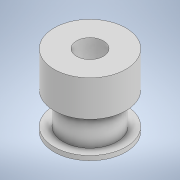
# Autodesk Inventor part: 20T pulley 6 mm bore GT2
Saved by Autodesk Inventor 2022 (Build 260153000, 153)
## iProperties
Created: 2022-08-12
Part Number: 20T pulley 6 mm bore GT2
Material: Genérico
Document SubType Name: Modeling
Designer: JK
Density: 1 g/cm^3
Appearance: Valor por defecto
Author: JK
Autodesk Inventor part; units mm, degrees
ref_plane "YZ Plane" through (0, 0, 0) normal (1, 0, 0) x (0, 1, 0)
ref_plane "XZ Plane" through (0, 0, 0) normal (0, 1, 0) x (-1, 0, 0)
ref_plane "XY Plane" through (0, 0, 0) normal (0, 0, 1) x (1, 0, 0)
sketch "Boceto1" plane through (0, 0, 0) normal (0, 1, 0) x (-1, 0, 0)
  circle A0 centre (0, 0) radius 8
  dimension "d0" = 16
  constraints: 1 centre point, 1 coincident
  measures "d0" diameter of A0
extrude "Extrusión1" add sketch "Boceto1" along normal blind 16
sketch "Boceto2" plane through (0, 16, 0) normal (0, 1, 0) x (1, 0, 0)
  circle A0 centre (0, 0) radius 3
  dimension "d3" = 6
  constraints: 1 centre point, 1 coincident
  measures "d3" diameter of A0
extrude "Extrusión2" cut sketch "Boceto2" against normal blind 16
sketch "Boceto3" plane through (0, 0, 0) normal (1, 0, 0) x (0, 1, 0)
  line L0 (0, 8) -> (16, 8) projected
  line L1 (1, 8) -> (8, 8)
  line L2 (8, 8) -> (8, 6)
  line L3 (8, 6) -> (1, 6)
  line L4 (1, 6) -> (1, 8)
  line L5 (16, -8) -> (16, 8) projected
  line L6 (0, -8) -> (0, 8) projected
  line L7 (0, 0) -> (16, 0)
  dimension "d6" = 2
  dimension "d7" = 7
  dimension "d8" = 1
  constraints: 10 end point, 2 horizontal, 2 midpoint, 2 parallel, 1 perpendicular, 1 point on line
  measures "d6" distance between parallel lines of L3 L0
  measures "d7" distance of L2.end L3.end
  measures "d8" distance between parallel lines of L4 L6
revolve "Revolución1" cut sketch "Boceto3" angle 360 about axis through (0, 0, 0) along (0, 1, 0) contours L0 L2 L3 L4
